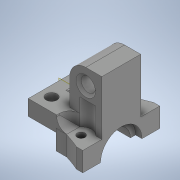
# Autodesk Inventor part: v6_Clamp V2
Saved by Autodesk Inventor 2022 (Build 260153000, 153)
## iProperties
Created: 2021-11-30
Part Number: v6_Clamp V2
Material: Polycarbonate, Clear
Document SubType Name: Modeling
Designer: alexr
Density: 1.2 g/cm^3
Appearance: Polycarbonate - Clear
Mass: 7.91539 g
Surface Area: 38.6835 cm^2
Volume: 6.59616 cm^3
Author: alexr
Autodesk Inventor part; units mm, degrees
ref_plane "YZ Plane" through (0, 0, 0) normal (1, 0, 0) x (0, 1, 0)
ref_plane "XZ Plane" through (0, 0, 0) normal (0, 1, 0) x (-1, 0, 0)
ref_plane "XY Plane" through (0, 0, 0) normal (0, 0, 1) x (1, 0, 0)
sketch "Sketch1" plane through (0, 0, 0) normal (0, 1, 0) x (-1, 0, 0)
  circle A0 centre (-13.0248, -40.295) radius 2 projected
  arc A1 (-16.0248, -35.532) -> (-10.0248, -37.7161) centre (4.9752, 12.8248) ccw projected
  line L0 (-16.0248, -35.532) -> (-18.4248, -35.532) projected
  line L1 (-18.4248, -42.245) -> (-18.4248, -35.532) projected
  line L2 (-16.0248, -42.245) -> (-18.4248, -42.245) projected
  line L3 (-16.0248, -44.295) -> (-16.0248, -42.245) projected
  line L4 (-10.0248, -44.295) -> (-16.0248, -44.295) projected
  line L5 (-10.0248, -42.245) -> (-10.0248, -44.295) projected
  line L6 (-10.0248, -42.245) -> (-6.0248, -42.245) projected
  line L7 (-6.0248, -37.7161) -> (-6.0248, -42.245) projected
  line L8 (-10.0248, -37.7161) -> (-6.0248, -37.7161) projected
  circle A2 centre (-13.0248, -60.495) radius 2 projected
  line L9 (-10.0248, -56.495) -> (-10.0248, -58.545) projected
  line L10 (-10.0248, -56.495) -> (-16.0248, -56.495) projected
  line L11 (-16.0248, -56.495) -> (-16.0248, -58.545) projected
  line L12 (-16.0248, -58.545) -> (-18.4248, -58.545) projected
  line L13 (-18.4248, -65.2581) -> (-18.4248, -58.545) projected
  line L14 (-16.0248, -65.2581) -> (-18.4248, -65.2581) projected
  arc A3 (-10.0248, -63.074) -> (-16.0248, -65.2581) centre (4.9752, -113.6149) ccw projected
  line L15 (-10.0248, -63.074) -> (-6.0248, -63.074) projected
  line L16 (-6.0248, -58.545) -> (-6.0248, -63.074) projected
  line L17 (-10.0248, -58.545) -> (-6.0248, -58.545) projected
  line L18 (-6.0248, -42.245) -> (-6.0248, -58.545)
  line L19 (-18.4248, -42.245) -> (-18.4248, -58.545)
  line L20 (-16.0248, -44.295) -> (-10.0248, -44.295)
  line L21 (-10.0248, -44.295) -> (-10.0248, -31.189)
  line L22 (-10.0248, -31.189) -> (-16.0248, -31.189)
  line L23 (-16.0248, -31.189) -> (-16.0248, -44.295)
  line L24 (-16.0248, -56.495) -> (-10.0248, -56.495)
  line L25 (-10.0248, -56.495) -> (-10.0248, -73.9089)
  line L26 (-10.0248, -73.9089) -> (-16.0248, -73.9089)
  line L27 (-16.0248, -73.9089) -> (-16.0248, -56.495)
  line L28 (-10.0248, -56.495) -> (-16.0248, -56.495)
  line L29 (-16.0248, -56.495) -> (-16.0248, -44.295)
  line L30 (-16.0248, -44.295) -> (-10.0248, -44.295)
  line L31 (-10.0248, -44.295) -> (-10.0248, -56.495)
  circle A4 centre (-13.0248, -40.295) radius 1.5
  circle A5 centre (-13.0248, -60.495) radius 1.5
  point P0 (0, 0)
  point P1 (-10.0248, -37.7161)
  dimension "d18" = 3
  dimension "d19" = 3
  constraints: 28 end point, 7 parallel, 3 horizontal, 3 perpendicular, 2 centre point, 2 coincident, 1 collinear, 1 point on line
  measures "d18" diameter of A4
  measures "d19" diameter of A5
extrude "Extrusion1" add sketch "Sketch1" along normal blind 11.5 contours A0 | A1 L21 L5 L4 L3 L23 | L4 L31 L10 L29 | L10 L9 L25 A3 L27 L11 | A2
sketch "Sketch2" plane through (10.0248, 0, -63.074) normal (-1, 0, 0) x (0, 0, 1)
  line L0 (0, 0) -> (25.3579, 0) projected
  circle A0 centre (12.6789, 0) radius 6.05
  point P0 (63.074, 0)
  dimension "d2" = 12.1
  constraints: 1 centre point, 1 midpoint
  measures "d2" diameter of A0
extrude "Extrusion2" cut sketch "Sketch2" against normal blind 11.5
sketch "Sketch3" plane through (10.0248, 0, -37.7161) normal (-1, 0, 0) x (0, 0, 1)
  circle A0 centre (27.6161, 0) radius 8 projected
  arc A1 (-6.6289, 0) -> (-18.7289, 0) centre (-12.6789, 0) ccw projected
  line L0 (-6.6289, 0) -> (0, 0) projected
  line L1 (0, 0) -> (0, 11.5) projected
  line L2 (-25.3579, 11.5) -> (0, 11.5) projected
  line L3 (-25.3579, 0) -> (-25.3579, 11.5) projected
  line L4 (-25.3579, 0) -> (-18.7289, 0) projected
  point P0 (37.7161, 0)
  point P1 (-20.6789, 0)
  point P2 (-4.6789, 0)
extrude "Extrusion3" add sketch "Sketch3" along normal blind 4 contours A1 L4 L3 L2 L1 L0
sketch "Sketch4" plane through (16.0248, 0, -65.2581) normal (1, 0, 0) x (0, 0, -1)
  circle A0 centre (-55.1581, 0) radius 8 projected
  arc A1 (-8.813, 0) -> (-20.913, 0) centre (-14.863, 0) ccw projected
  line L0 (-8.813, 0) -> (0, 0) projected
  line L1 (0, 0) -> (0, 11.5) projected
  line L2 (-29.726, 11.5) -> (0, 11.5) projected
  line L3 (-29.726, 0) -> (-29.726, 11.5) projected
  line L4 (-29.726, 0) -> (-20.913, 0) projected
  point P0 (-65.2581, 0)
  point P1 (-22.863, 0)
  point P2 (-6.863, 0)
extrude "Extrusion4" add sketch "Sketch4" along normal blind 2.4 contours A1 L4 L3 L2 L1 L0
sketch "Sketch5" plane through (0, 11.5, 0) normal (0, 1, 0) x (1, 0, 0)
  arc A0 (10.0248, 63.074) -> (16.0248, 65.2581) centre (-4.9752, 113.6149) ccw projected
  line L0 (10.0248, 63.074) -> (6.0248, 63.074) projected
  line L1 (6.0248, 37.7161) -> (6.0248, 63.074) projected
  line L2 (10.0248, 37.7161) -> (6.0248, 37.7161) projected
  arc A1 (16.0248, 35.532) -> (10.0248, 37.7161) centre (-4.9752, -12.8248) ccw projected
  line L3 (16.0248, 35.532) -> (18.4248, 35.532) projected
  line L4 (18.4248, 65.2581) -> (18.4248, 35.532) projected
  line L5 (16.0248, 65.2581) -> (18.4248, 65.2581) projected
  line L6 (18.4248, 65.2581) -> (18.4248, 35.532) projected
  line L7 (6.0248, 42.895) -> (18.4248, 42.895)
  line L8 (18.4248, 42.895) -> (18.4248, 57.895)
  line L9 (18.4248, 57.895) -> (6.0248, 57.895)
  line L10 (6.0248, 57.895) -> (6.0248, 42.895)
  point P0 (0, 0)
  point P1 (6.0248, 57.895)
  point P2 (18.4248, 42.895)
  dimension "d9" = 15
  constraints: 8 end point, 2 parallel, 2 point on line, 1 horizontal, 1 perpendicular
  measures "d9" distance of L8.end L7.end
extrude "Extrusion5" add sketch "Sketch5" along normal blind 17 contours L9 L4 L7 L1
sketch "Sketch6" plane through (0, 11.5, 0) normal (0, 1, 0) x (1, 0, 0)
  circle A0 centre (13.0248, 40.295) radius 2 projected
  circle A1 centre (13.0248, 40.295) radius 4
  circle A2 centre (13.0248, 60.495) radius 2 projected
  circle A3 centre (13.0248, 60.495) radius 4
  point P0 (0, 0)
  dimension "d14" = 8
  dimension "d15" = 8
  constraints: 2 centre point, 2 coincident
  measures "d14" diameter of A1
  measures "d15" diameter of A3
extrude "Extrusion6" cut sketch "Sketch6" along normal blind 6 contours A1 | A2 | A3
sketch "Sketch7" plane through (6.0248, 28.5, -42.895) normal (0, 0, 1) x (1, 0, 0)
  circle A0 centre (6.2, -6.2) radius 2.75
  line L0 (0, -17) -> (0, 0) projected
  line L1 (12.4, -17) -> (12.4, 0) projected
  line L2 (0, 0) -> (12.4, 0) projected
  point P0 (-6.0248, -28.5)
  dimension "d20" = 5.5
  dimension "d21" = 12.4
  dimension "d23" = 6.2
  dimension "d24" = 6.2
  constraints: 1 centre point
  measures "d20" diameter of A0
  measures "d21" distance between parallel lines of L0 L1
  measures "d23" distance from line of L0 A0.centre
  measures "d24" distance from line of L2 A0.centre
extrude "Extrusion7" cut sketch "Sketch7" against normal blind 27.25
sketch "Sketch8" plane through (18.4248, 28.5, -57.895) normal (0, 0, -1) x (-1, 0, 0)
  circle A0 centre (6.2, -6.2) radius 2.75 projected
  circle A1 centre (6.2, -6.2) radius 4.1
  circle A2 centre (6.2, -6.2) radius 2.75 projected
  line L0 (8.4397, -11) -> (8.4397, -17) projected
  line L1 (12.4, -17) -> (8.4397, -17) projected
  line L2 (12.4, -17) -> (12.4, 0) projected
  line L3 (0, 0) -> (12.4, 0) projected
  line L4 (0, -17) -> (0, 0) projected
  line L5 (2.3603, -17) -> (0, -17) projected
  line L6 (2.3603, -17) -> (2.3603, -11) projected
  line L7 (2.3603, -11) -> (8.4397, -11) projected
  line L8 (12.4, -17) -> (12.4, 0) projected
  line L9 (0, -17) -> (0, 0) projected
  line L10 (12.4, 0) -> (0, 0)
  line L11 (0, 0) -> (0, -11)
  line L12 (0, -11) -> (12.4, -11)
  line L13 (12.4, -11) -> (12.4, 0)
  point P0 (18.4248, -28.5)
  dimension "d27" = 8.2
  constraints: 8 end point, 2 parallel, 1 centre point, 1 coincident, 1 horizontal, 1 perpendicular, 1 point on line
  measures "d27" diameter of A1
sketch "Sketch9" plane through (0, 11.5, 0) normal (0, 1, 0) x (1, 0, 0)
  line L0 (9.985, 42.895) -> (6.0248, 42.895) projected
  line L1 (6.0248, 37.7161) -> (6.0248, 42.895) projected
  line L2 (10.0248, 37.7161) -> (6.0248, 37.7161) projected
  arc A0 (16.0248, 35.532) -> (10.0248, 37.7161) centre (-4.9752, -12.8248) ccw projected
  line L3 (16.0248, 35.532) -> (18.4248, 35.532) projected
  line L4 (18.4248, 42.895) -> (18.4248, 35.532) projected
  line L5 (18.4248, 42.895) -> (16.0645, 42.895) projected
  arc A1 (16.0645, 42.895) -> (9.985, 42.895) centre (13.0248, 40.295) ccw projected
  circle A2 centre (13.0248, 40.295) radius 1.5 projected
  circle A3 centre (13.0248, 60.495) radius 1.5 projected
  line L6 (10.0248, 63.074) -> (6.0248, 63.074) projected
  line L7 (6.0248, 57.895) -> (6.0248, 63.074) projected
  line L8 (6.0248, 57.895) -> (9.985, 57.895) projected
  arc A4 (9.985, 57.895) -> (16.0645, 57.895) centre (13.0248, 60.495) ccw projected
  line L9 (16.0645, 57.895) -> (18.4248, 57.895) projected
  line L10 (18.4248, 65.2581) -> (18.4248, 57.895) projected
  line L11 (16.0248, 65.2581) -> (18.4248, 65.2581) projected
  arc A5 (10.0248, 63.074) -> (16.0248, 65.2581) centre (-4.9752, 113.6149) ccw projected
  point P0 (0, 0)
extrude "Extrusion8" cut sketch "Sketch9" against normal blind 4
extrude "Extrusion9" [suppressed]
fillet "Fillet1" [suppressed]
sketch "Sketch10" plane through (6.0248, 0, -37.7161) normal (-1, 0, 0) x (0, 0, 1)
  line L0 (-5.3531, 14.25) -> (-5.4408, 14.25) projected
  line L1 (-34.4289, 6) -> (9.0711, 6) projected
  line L2 (-20.1789, 28.5) -> (-20.1789, 7.5) projected
  line L3 (-5.1789, 6) -> (-20.1789, 6)
  line L4 (-20.1789, 6) -> (-20.1789, 12)
  line L5 (-20.1789, 12) -> (-5.1789, 12)
  line L6 (-5.1789, 12) -> (-5.1789, 6)
  line L7 (-5.1789, 12) -> (-0.1789, 12)
  line L8 (-0.1789, 12) -> (-0.1789, 6)
  line L9 (-0.1789, 6) -> (-5.1789, 6)
  line L10 (-5.1789, 6) -> (-5.1789, 12)
  line L11 (-20.1789, 12) -> (-25.1789, 12)
  line L12 (-25.1789, 12) -> (-25.1789, 6)
  line L13 (-25.1789, 6) -> (-20.1789, 6)
  line L14 (-20.1789, 6) -> (-20.1789, 12)
  point P0 (37.7161, 0)
  point P1 (-20.1789, 17.5)
  point P2 (-20.1789, 7.5)
  dimension "d33" = 6
  dimension "d48" = 5
  dimension "d49" = 5
  constraints: 24 end point, 6 parallel, 4 point on line, 3 horizontal, 3 perpendicular
  measures "d33" distance of L3.end L4.end
  measures "d48" distance of L8.end L9.end
  measures "d49" distance of L13.end L12.end
extrude "Extrusion10" add sketch "Sketch10" along normal blind 11
chamfer "Chamfer1" distance 1 angle 45 1 edges at (9.4748, 22.3, -42.895)
sketch "Sketch12" plane through (6.0248, 12, -37.895) normal (0, 1, 0) x (1, 0, 0)
  line L0 (-3, -15.25) -> (-3, -9.25) projected
  line L1 (-11, -9.25) -> (-11, -15.25) projected
  circle A0 centre (-7, 5) radius 2.1
  line L2 (0, 0) -> (-11, 0) projected
  line L3 (-11, 25) -> (-11, 0) projected
  line L4 (-11, 12.5) -> (-8.4251, 12.5)
  circle A1 centre (-7, 20) radius 2.1
  point P0 (-6.0248, -37.895)
  dimension "d50" = 8
  dimension "d51" = 4.2
  dimension "d52" = 4
  dimension "d53" = 5
  constraints: 2 centre point, 2 end point, 1 horizontal, 1 midpoint, 1 symmetric about line, 1 other
  measures "d50" distance from line of L1.end L0
  measures "d51" diameter of A0
  measures "d52" distance from line of A0.centre L0
  measures "d53" distance from line of L2 A0.centre
extrude "Extrusion12" cut sketch "Sketch12" against normal blind 11
fillet "Fillet2" radius 3.9 4 edges at (6.0248, 9.75, -42.895) (6.0248, 7.5, -40.395) (6.0248, 9.75, -57.895) (6.0248, 7.5, -60.395)
sketch "Sketch13" plane through (6.0248, 0, -37.7161) normal (-1, 0, 0) x (0, 0, 1)
  circle A0 centre (-12.6789, 0) radius 8 projected
  point P0 (37.7161, 0)
extrude "Extrusion13" cut sketch "Sketch13" against normal blind 4
sketch "Sketch14" plane through (18.4248, 0, -65.2581) normal (1, 0, 0) x (0, 0, -1)
  arc A0 (-23.013, 0) -> (-6.713, 0) centre (-14.863, 0) ccw projected
  circle A1 centre (-14.863, 0) radius 8 projected
  point P0 (-65.2581, 0)
extrude "Extrusion14" cut sketch "Sketch14" against normal blind 2.5
fillet "Fillet3" radius 6.2 1 edges at (6.0248, 28.5, -50.395)
ref_plane "Work Plane1" through (6.0248, 6, -50.395) normal (0, 0, -1) x (-1, 0, 0)
sketch "Sketch15" plane through (6.0248, 6, -50.395) normal (0, 0, -1) x (-1, 0, 0)
  line L0 (0, 16.3) -> (0, 6) projected
  line L1 (0, 6) -> (11, 6) projected
  arc A0 (0, 16.3) -> (-6.2, 22.5) centre (-6.2, 16.3) ccw projected
  line L2 (0, 16.3) -> (0, 16.3)
  line L3 (6.5, 6) -> (11, 6)
  line L4 (0, 6) -> (4.5, 6)
  line L5 (4.5, 8) -> (4.5, 12.3)
  line L6 (2.5, 14.3) -> (2, 14.3)
  line L7 (0, 14.3) -> (0, 6)
  arc A1 (0, 16.3) -> (2, 14.3) centre (2, 16.3) ccw
  arc A2 (4.5, 12.3) -> (2.5, 14.3) centre (2.5, 12.3) ccw
  line L8 (0, 6) -> (0, 16.3) projected
  line L9 (0, 12) -> (1.5, 12)
  line L10 (2.5, 11) -> (2.5, 6)
  line L11 (2.5, 6) -> (0, 6)
  line L12 (0, 6) -> (0, 12)
  arc A3 (4.5, 8) -> (6.5, 6) centre (6.5, 8) ccw
  arc A4 (2.5, 11) -> (1.5, 12) centre (1.5, 11) ccw
  point P0 (6.0248, -6)
  point P1 (4.5, 14.3)
  point P2 (0, 16.3)
  point P3 (6.5, 6)
  dimension "d64" = 2
  dimension "d66" = 2
  dimension "d67" = 2.5
  dimension "d68" = 2
  dimension "d69" = 1
  dimension "d70" = 6
  dimension "d73" = 2
  dimension "d75" = 0
  constraints: 20 end point, 8 point on circle, 8 point on line, 8 tangent, 4 centre point, 4 parallel, 2 horizontal, 2 perpendicular, 1 collinear
  measures "d64" radius of A1
  measures "d66" radius of A2
  measures "d67" distance of L10.end L11.end
  measures "d68" radius of A3
  measures "d69" radius of A4
  measures "d70" distance between parallel lines of L11 L9
  measures "d73" distance between parallel lines of L5 L10
  measures "d75" distance of L0.start L2.end
extrude "Extrusion15" add sketch "Sketch15" along normal mid plane 4 contours A1 L6 A2 L5 A3 L1 L10 A4 L9 L0
chamfer "Chamfer3" distance 0.5 angle 45 10 edges at (3.5248, 14.5, -52.395) (3.8176, 17.7071, -52.395) (5.2748, 18, -52.395) (3.8176, 17.7071, -48.395) (5.2748, 18, -48.395) (3.5248, 14.5, -48.395) (6.0248, 20.15, -48.395) (6.0248, 20.15, -52.395) (1.5248, 12, -52.395) (1.5248, 12, -48.395)
equation "\"d15\" = d14"
equation "\"d23\" = 0.5 * d21"
equation "\"d24\" = d23"
equation "\"d52\" = 0.5 * d50"
equation "\"d66\" = d64"
body "Solid1"
